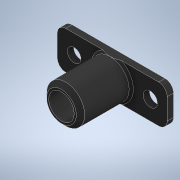
# Autodesk Inventor part: LightSensorHolder
Saved by Autodesk Inventor 2021 (Build 250183000, 183)
## iProperties
Created: 2020-07-16
Part Number: LightSensorHolder
Material: Generic
Document SubType Name: Modeling
Designer: CASE-SMALL2
Density: 1 g/cm^3
Appearance: Default
Author: CASE-SMALL2
Autodesk Inventor part; units mm, degrees
ref_plane "YZ Plane" through (0, 0, 0) normal (1, 0, 0) x (0, 1, 0)
ref_plane "XZ Plane" through (0, 0, 0) normal (0, 1, 0) x (-1, 0, 0)
ref_plane "XY Plane" through (0, 0, 0) normal (0, 0, 1) x (1, 0, 0)
sketch "Sketch1" plane through (0, 0, 0) normal (0, 0, 1) x (1, 0, 0)
  circle A0 centre (0, 0) radius 3
  circle A1 centre (0, 0) radius 4.5
  dimension "d0" = 6
  dimension "d1" = 1.5
  constraints: 2 centre point, 2 coincident
  measures "d0" diameter of A0
  measures "d1" radial gap between concentric circles of A1 A0
extrude "Extrusion1" add sketch "Sketch1" along normal blind 4
sketch "Sketch2" plane through (0, 0, 4) normal (0, 0, 1) x (1, 0, 0)
  circle A0 centre (0, 0) radius 4.5 projected
  line L0 (-6.3, 0) -> (6.3, 0) construction
  circle A1 centre (-1.5, 0) radius 0.75
  circle A2 centre (1.5, 0) radius 0.8535
  dimension "d4" = 1.5
  dimension "d5" = 1.5
  dimension "d6" = 1.5
  constraints: 2 centre point, 2 point on line
  measures "d4" diameter of A1
  measures "d5" distance of point (0, 0) A1.centre
  measures "d6" distance of point (0, 0) A2.centre
extrude "Extrusion2" add sketch "Sketch2" along normal blind 1.5
sketch "Sketch3" plane through (0, 0, 0) normal (0, 0, -1) x (-1, 0, 0)
  line L0 (-13, 4.5) -> (13, 4.5)
  line L1 (13, 4.5) -> (13, -4.5)
  line L2 (13, -4.5) -> (-13, -4.5)
  line L3 (-13, -4.5) -> (-13, 4.5)
  line L4 (-13, 4.5) -> (13, -4.5) construction
  line L5 (13, 4.5) -> (-13, -4.5) construction
  circle A0 centre (0, 0) radius 4.5 projected
  point P0 (0, -4.5)
  point P1 (0, 4.5)
  dimension "d9" = 26
  constraints: 12 end point, 2 midpoint, 2 parallel, 1 horizontal, 1 perpendicular, 1 tangent
  measures "d9" distance of L1.end L2.end
extrude "Extrusion3" add sketch "Sketch3" against normal blind 1.5 contours L0 A0 L2 L3 | L0 L1 L2 A0
fillet "Fillet1" radius 2 4 edges at (13, 4.5, 0.75) (13, -4.5, 0.75) (-13, 4.5, 0.75) (-13, -4.5, 0.75)
sketch "Sketch4" plane through (0, 0, 0) normal (0, 0, -1) x (-1, 0, 0)
  line L0 (18.2, 0) -> (-18.2, 0) projected
  circle A0 centre (9, 0) radius 1.5974
  circle A1 centre (-9, 0) radius 1.6824
  point P0 (0, 0)
  dimension "d13" = 9
  dimension "d14" = 9
  constraints: 2 centre point, 2 point on line
  measures "d13" distance of point (0, 0) A0.centre
  measures "d14" distance of point (0, 0) A1.centre
extrude "Extrusion4" cut sketch "Sketch4" against normal through all
chamfer "Chamfer1" distance 0.5 angle 45 3 edges at (3.182, 3.182, 1.5) (3.182, -3.182, 1.5) (-4.5, 0, 1.5)
sketch "Sketch5" plane through (0, 0, 5.5) normal (0, 0, 1) x (1, 0, 0)
  circle A0 centre (0, 0) radius 4.5 projected
  circle A1 centre (0, 0) radius 3 projected
extrude "Extrusion5" add sketch "Sketch5" along normal blind 8
chamfer "Chamfer2" distance 1 angle 45 1 edges at (-4.5, 0, 13.5)
equation "\"d6\" = d5"
equation "\"d14\" = d13"
body "Solid1"
